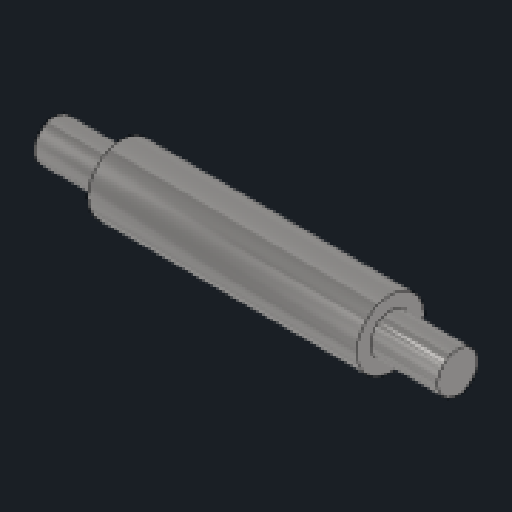
# Autodesk Inventor part: Pin
Saved by Autodesk Inventor 2023.2 (Build 272271030, 271C)
## iProperties
Created: 2024-02-21
Part Number: Pin
Material: Stainless Steel
Document SubType Name: Modeling
Designer: robpl
Density: 8 g/cm^3
Appearance: Semi-Polished
Mass: 1.90015 g
Surface Area: 3.15071 cm^2
Volume: 0.237519 cm^3
Author: robpl
Autodesk Inventor part; units mm, degrees
ref_plane "YZ Plane" through (0, 0, 0) normal (1, 0, 0) x (0, 1, 0)
ref_plane "XZ Plane" through (0, 0, 0) normal (0, 1, 0) x (-1, 0, 0)
ref_plane "XY Plane" through (0, 0, 0) normal (0, 0, 1) x (1, 0, 0)
sketch "Sketch2" plane through (0, 0, 0) normal (0, 0, 1) x (1, 0, 0)
  line L0 (-15, 0) -> (15, 0)
  line L1 (15, 0) -> (15, 2.5)
  line L2 (15, 2.5) -> (-15, 2.5)
  line L3 (-15, 2.5) -> (-15, 0)
  line L4 (15, 2.5) -> (10, 2.5)
  line L5 (10, 2.5) -> (10, 1.5)
  line L6 (10, 1.5) -> (15, 1.5)
  line L7 (15, 1.5) -> (15, 2.5)
  line L8 (-15, 2.5) -> (-10, 2.5)
  line L9 (-10, 2.5) -> (-10, 1.5)
  line L10 (-10, 1.5) -> (-15, 1.5)
  line L11 (-15, 1.5) -> (-15, 2.5)
  point P0 (0, 0)
  point P1 (0, 0)
  dimension "d3" = 30
  dimension "d4" = 2.5
  dimension "d5" = 1.5
  dimension "d6" = 5
  constraints: 24 end point, 6 parallel, 3 horizontal, 3 perpendicular, 2 equal length, 1 coincident, 1 midpoint
  measures "d3" distance of L1.end L2.end
  measures "d4" distance of L0.end L1.end
  measures "d5" distance between parallel lines of L0 L6
  measures "d6" distance of L5.end L6.end
revolve "Revolution1" add sketch "Sketch2" angle 360 about axis through (-15, 0, 0) along (1, 0, 0) contours L3 L10 L9 L2 L5 L6 L1 L0
body "Solid2"
